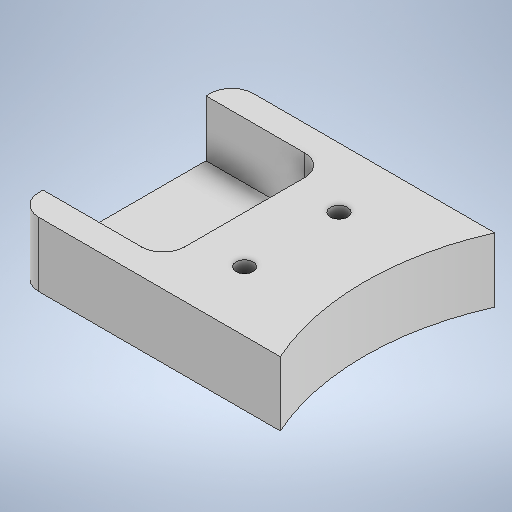
# Autodesk Inventor part: Head Plate Inserts
Saved by Autodesk Inventor 2025 (Build 290162000, 162)
## iProperties
Created: 2025-06-24
Part Number: Head Plate Inserts
Material: Generic
Document SubType Name: Modeling
Designer: mumin
Density: 1 g/cm^3
Appearance: Default
Author: mumin
Autodesk Inventor part; units mm, degrees
ref_plane "YZ Plane" through (0, 0, 0) normal (1, 0, 0) x (0, 1, 0)
ref_plane "XZ Plane" through (0, 0, 0) normal (0, 1, 0) x (-1, 0, 0)
ref_plane "XY Plane" through (0, 0, 0) normal (0, 0, 1) x (1, 0, 0)
sketch "Sketch1" plane through (0, 0, 0) normal (0, 1, 0) x (-1, 0, 0)
  circle A0 centre (0, 0) radius 42.5
  arc A1 (55.6417, 25) -> (-59.6645, -12.6946) centre (0, 0) ccw
  line L0 (0, 0) -> (0, -61)
  line L1 (0, 0) -> (0, 0)
  line L2 (117.5, -25) -> (117.5, 25)
  line L3 (117.5, 25) -> (-117.5, -25) construction
  line L4 (-117.5, 25) -> (117.5, -25) construction
  line L5 (117.5, 25) -> (55.6417, 25)
  line L6 (55.6417, -25) -> (117.5, -25)
  arc A2 (-59.6645, -12.6946) -> (55.6417, -25) centre (0, 0) ccw
  point P0 (0, -61)
  point P1 (-59.6645, 12.6946)
  dimension "d0" = 85
  dimension "d1" = 61
  dimension "d2" = 235
  constraints: 14 end point, 5 coincident, 5 point on circle, 3 centre point, 2 horizontal, 2 midpoint, 2 point on line, 1 parallel, 1 vertical, 1 vertical alignment
  measures "d0" diameter of A0
  measures "d1" radius of A1
  measures "d2" distance of L4.end L3.end
extrude "Head Plate Geometry" add sketch "Sketch1" along normal blind 15
sketch "Sketch2" plane through (0, 15, 0) normal (0, 1, 0) x (1, 0, 0)
  line L0 (-117.5, 25) -> (-117.5, -25) projected
  line L1 (-117.5, 19) -> (-94.5, 19)
  line L2 (-89.5, 14) -> (-89.5, -14)
  line L3 (-94.5, -19) -> (-117.5, -19)
  arc A0 (-89.5, 14) -> (-94.5, 19) centre (-94.5, 14) ccw
  arc A1 (-94.5, -19) -> (-89.5, -14) centre (-94.5, -14) ccw
  line L4 (-117.5, 25) -> (-117.5, -25) projected
  line L5 (-153.2, 0) -> (96.7, 0) projected
  point P0 (0, 0)
  dimension "d6" = 5
  dimension "d7" = 38
  dimension "d8" = 28
  constraints: 6 end point, 4 point on circle, 4 tangent, 2 centre point, 2 perpendicular, 2 point on line, 1 equal radius, 1 horizontal, 1 other
  measures "d6" radius of A0
  measures "d7" distance between parallel lines of L3 L1
  measures "d8" distance between parallel lines of L2 L0
extrude "Magnet Seat" cut sketch "Sketch2" against normal blind 13.1
sketch "Sketch3" plane through (0, 0, 0) normal (0, -1, 0) x (1, 0, 0)
  line L0 (-117.5, -25) -> (-117.5, 25) projected
  line L1 (-153.2, 0) -> (96.7, 0) projected
  point P0 (0, 0)
  point P1 (-78.5, -11)
  point P2 (-78.5, 11)
  dimension "d19" = 39
  dimension "d22" = 11
  constraints: 1 symmetric about line
  measures "d19" distance from line of L0 point (-78.5, -11)
  measures "d22" distance from line of L1 point (-78.5, -11)
hole "Hole1" at (-78.5, 0, -11) at (-78.5, 0, 11) direction (0, 1, 0) diameter 4 depth 15 counterbore diameter 8 counterbore depth 6
fillet "Fillet1" radius 5 2 edges at (-117.5, 7.5, -25) (-117.5, 7.5, 25)
sketch "Sketch4" plane through (0, 0, 0) normal (0, -1, 0) x (1, 0, 0)
  circle A0 centre (0, 0) radius 61.5
  dimension "d24" = 123
  constraints: 1 centre point, 1 coincident
  measures "d24" diameter of A0
extrude "Remove Material" cut sketch "Sketch4" against normal through all
body "Solid1"
